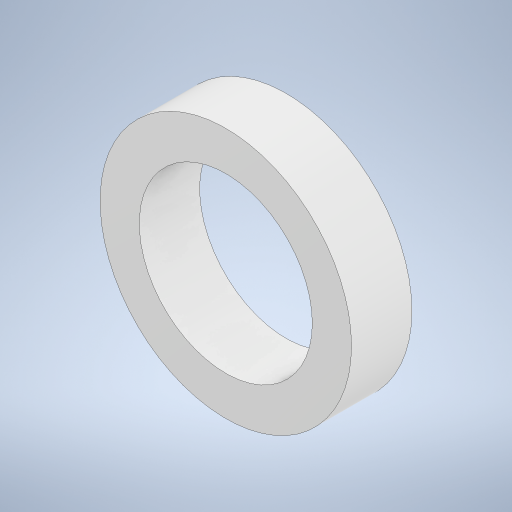
# Autodesk Inventor part: Door Bar Bearing Door Mounting Spacer
Saved by Autodesk Inventor 2024 (Build 280153000, 153)
## iProperties
Created: 2024-08-29
Part Number: Door Bar Bearing Door Mounting Spacer
Material: ABS Plastic
Document SubType Name: Modeling
Designer: Ishaan
Density: 1.06 g/cm^3
Appearance: Smooth - White
Author: Ishaan
Autodesk Inventor part; units mm, degrees
ref_plane "YZ Plane" through (0, 0, 0) normal (1, 0, 0) x (0, 1, 0)
ref_plane "XZ Plane" through (0, 0, 0) normal (0, 1, 0) x (-1, 0, 0)
ref_plane "XY Plane" through (0, 0, 0) normal (0, 0, 1) x (1, 0, 0)
sketch "Sketch1" plane through (0, 0, 0) normal (0, 0, 1) x (1, 0, 0)
  circle A0 centre (0, 0) radius 2.65
  circle A1 centre (0, 0) radius 3.85
  dimension "d0" = 5.3
  dimension "d1" = 1.2
  constraints: 2 centre point, 2 coincident
  measures "d0" diameter of A0
  measures "d1" radial gap between concentric circles of A1 A0
extrude "Extrusion1" add sketch "Sketch1" along normal blind 1.85
body "Solid1"
